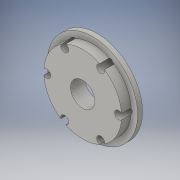
# Autodesk Inventor part: Part1
Saved by Autodesk Inventor 2016 (Build 200138000, 138)
## iProperties
Created: 2016-02-19
Part Number: Part1
Material: Generic
Document SubType Name: Modeling
Designer: RoksBot
Density: 1 g/cm^3
Appearance: Default
Author: RoksBot
Autodesk Inventor part; units mm, degrees
ref_plane "YZ Plane" through (0, 0, 0) normal (1, 0, 0) x (0, 1, 0)
ref_plane "XZ Plane" through (0, 0, 0) normal (0, 1, 0) x (-1, 0, 0)
ref_plane "XY Plane" through (0, 0, 0) normal (0, 0, 1) x (1, 0, 0)
sketch "Sketch1" plane through (0, 0, 0) normal (0, 0, 1) x (1, 0, 0)
  circle A0 centre (0, 0) radius 25.7048
  dimension "d0" = 51.4096
  constraints: 1 centre point, 1 coincident
  measures "d0" diameter of A0
extrude "Extrusion1" add sketch "Sketch1" along normal blind 6.4262
sketch "Sketch2" plane through (0, 0, 6.4262) normal (0, 0, 1) x (1, 0, 0)
  circle A0 centre (0, 0) radius 8.0645
  dimension "d3" = 16.129
  constraints: 1 centre point, 1 coincident
  measures "d3" diameter of A0
extrude "Extrusion2" cut sketch "Sketch2" against normal blind 127
sketch "Sketch3" plane through (0, 0, 0) normal (0, 0, -1) x (-1, 0, 0)
  circle A0 centre (0, 0) radius 29.9085
  dimension "d6" = 59.817
  constraints: 1 centre point, 1 coincident
  measures "d6" diameter of A0
extrude "Extrusion3" add sketch "Sketch3" along normal blind 3.2512
sketch "Sketch4" plane through (0, 0, 6.4262) normal (0, 0, 1) x (1, 0, 0)
  circle A0 centre (0, 0) radius 8.0645
  constraints: 1 centre point, 1 coincident
extrude "Extrusion4" cut sketch "Sketch4" against normal blind 127
sketch "Sketch5" plane through (0, 0, -3.2512) normal (0, 0, -1) x (-1, 0, 0)
  circle A0 centre (23.7744, 0) radius 2.6416
  circle A1 centre (-23.7744, 0) radius 2.6416
  circle A2 centre (0, 0) radius 29.9085 projected
  circle A3 centre (0, 0) radius 8.0645 projected
  line L0 (0, 8.0645) -> (0, -8.0645) construction
  dimension "d11" = 5.2832
  dimension "d12" = 42.2656
  constraints: 2 centre point, 2 end point, 2 horizontal alignment, 2 point on circle, 1 equal radius, 1 midpoint, 1 vertical, 1 other
  measures "d11" diameter of A0
extrude "Extrusion5" cut sketch "Sketch5" against normal through all contours A0 | A1
pattern_circular "Circular Pattern1" count 3 over 360 about axis through (0, 0, 6.4262) along (0, 0, -1) of "Extrusion5"
body "Solid1"
